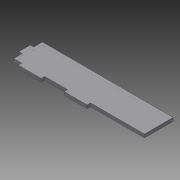
# Autodesk Inventor part: motor reinforcment
Saved by Autodesk Inventor 2015 (Build 190159000, 159)
## iProperties
Created: 2014-08-15
Part Number: motor reinforcment
Material: Generic
Document SubType Name: Modeling
Designer: karl
Density: 1 g/cm^3
Appearance: Default
Author: karl
Autodesk Inventor part; units mm, degrees
ref_plane "YZ Plane" through (0, 0, 0) normal (1, 0, 0) x (0, 1, 0)
ref_plane "XZ Plane" through (0, 0, 0) normal (0, 1, 0) x (-1, 0, 0)
ref_plane "XY Plane" through (0, 0, 0) normal (0, 0, 1) x (1, 0, 0)
sketch "Sketch1" plane through (0, 0, 0) normal (0, 0, 1) x (1, 0, 0)
  line L0 (57, -12.5) -> (-57, -12.5)
  line L1 (-57, -12.5) -> (-57, 12.5)
  line L2 (-57, 12.5) -> (57, 12.5)
  line L3 (57, 12.5) -> (57, -12.5)
  line L4 (57, -12.5) -> (-57, 12.5) construction
  line L5 (-57, -12.5) -> (57, 12.5) construction
  point P0 (0, 0)
  dimension "d0" = 57
  dimension "d1" = 25
  constraints: 12 end point, 2 midpoint, 2 parallel, 1 horizontal, 1 perpendicular
  measures "d0" distance from line of L1 point (0, 0)
  measures "d1" distance between parallel lines of L0 L2
extrude "Extrusion1" add sketch "Sketch1" along normal blind 3
sketch "Sketch2" plane through (0, 0, 0) normal (0, 0, -1) x (-1, 0, 0)
  line L0 (57, 12.5) -> (57, -12.5) projected
  line L1 (57, 5) -> (60, 5)
  line L2 (60, 5) -> (60, -5)
  line L3 (60, -5) -> (57, -5)
  line L4 (57, -5) -> (57, 5)
  point P0 (0, 0)
  point P1 (60, 0)
  dimension "d4" = 3
  dimension "d5" = 10
  constraints: 8 end point, 2 parallel, 1 horizontal, 1 horizontal alignment, 1 midpoint, 1 perpendicular, 1 point on line
  measures "d4" distance of L2.end L3.end
  measures "d5" distance of L1.end L2.end
extrude "Extrusion2" add sketch "Sketch2" against normal blind 3
sketch "Sketch3" plane through (0, 0, 0) normal (0, 0, -1) x (-1, 0, 0)
  line L0 (-57, -12.5) -> (57, -12.5) projected
  line L1 (50, -12.5) -> (30, -12.5)
  line L2 (30, -12.5) -> (30, -15.5)
  line L3 (30, -15.5) -> (50, -15.5)
  line L4 (50, -15.5) -> (50, -12.5)
  line L5 (-10, -12.5) -> (10, -12.5)
  line L6 (10, -12.5) -> (10, -15.5)
  line L7 (10, -15.5) -> (-10, -15.5)
  line L8 (-10, -15.5) -> (-10, -12.5)
  point P0 (0, 0)
  point P1 (0, -15.5)
  dimension "d8" = 20
  dimension "d9" = 3
  dimension "d10" = 30
  dimension "d11" = 20
  dimension "d12" = 3
  dimension "d13" = 20
  constraints: 16 end point, 4 parallel, 2 horizontal, 2 perpendicular, 2 point on line, 1 midpoint, 1 vertical alignment
  measures "d8" distance of L3.end L2.end
  measures "d9" distance of L2.end L1.end
  measures "d10" distance from line of L2 point (0, 0)
  measures "d11" distance of L6.end L7.end
  measures "d12" distance of L5.end L6.end
  measures "d13" distance between parallel lines of L2 L6
extrude "Extrusion3" add sketch "Sketch3" against normal blind 3
body "Solid1"
